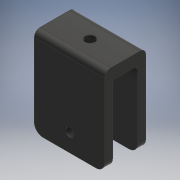
# Autodesk Inventor part: Y_Idler
Saved by Autodesk Inventor 2017.3 (Build 213256000, 256)
## iProperties
Created: 2018-09-09
Part Number: Y_Idler
Material: ABS Plastic
Document SubType Name: Modeling
Designer: Ax
Density: 1.06 g/cm^3
Appearance: Smooth - Black
Author: Ax
## iProperties of the stored document Y_Idler_3DPrint.ipt
Created: 2018-09-09
Part Number: Y_Idler_3DPrint
Material: Generic
Document SubType Name: Modeling
Designer: Ax
Density: 1 g/cm^3
Appearance: Default
Author: Ax
Autodesk Inventor part; units mm, degrees
ref_plane "YZ Plane" through (0, 0, 0) normal (1, 0, 0) x (0, 1, 0)
ref_plane "XZ Plane" through (0, 0, 0) normal (0, 1, 0) x (-1, 0, 0)
ref_plane "XY Plane" through (0, 0, 0) normal (0, 0, 1) x (1, 0, 0)
sketch "Sketch1" plane through (0, 0, 0) normal (1, 0, 0) x (0, 1, 0)
  line L0 (7, -26) -> (7, 4)
  line L1 (7, 4) -> (-7, 4)
  line L2 (-7, 4) -> (-7, -26)
  line L3 (-7, -26) -> (-4.25, -26)
  line L4 (-4.25, -26) -> (-4.25, 0)
  line L5 (-4.25, 0) -> (4.25, 0)
  line L6 (4.25, 0) -> (4.25, -26)
  line L7 (4.25, -26) -> (7, -26)
  line L8 (0, 0) -> (0, 4) construction
  dimension "d0" = 8.5
  dimension "d1" = 30
  dimension "d2" = 4
  dimension "d4" = 14
  constraints: 18 end point, 6 perpendicular, 2 equal length, 2 midpoint, 2 vertical, 1 coincident, 1 symmetric about line
  measures "d0" distance of L4.end L5.end
  measures "d1" distance of L0.start L0.end
  measures "d2" vertical distance of L0.end L5.end
  measures "d4" distance of L2.end L0.start
extrude "Extrusion1" add sketch "Sketch1" along normal mid plane 24
sketch "Sketch2" plane through (-12, 7, 4) normal (0, 1, 0) x (1, 0, 0)
  line L0 (12, 30) -> (12, 0) construction
  line L1 (24, 30) -> (0, 30) construction
  line L2 (0, 0) -> (24, 0) construction
  circle A0 centre (12, 24) radius 1.5
  point P0 (12, 4)
  dimension "d7" = 3
  dimension "d8" = 6
  constraints: 2 end point, 2 midpoint, 1 centre point, 1 point on line, 1 vertical
  measures "d7" diameter of A0
  measures "d8" distance of L0.start A0.centre
extrude "Extrusion2" cut sketch "Sketch2" against normal through all
sketch "Sketch3" plane through (-12, -7, 4) normal (0, 0, 1) x (1, 0, 0)
  circle A0 centre (12, 7) radius 1.7
  dimension "d11" = 3.4
  constraints: 1 centre point, 1 coincident
  measures "d11" diameter of A0
extrude "Extrusion3" cut sketch "Sketch3" against normal up to surface (4 mm away)
sketch "Sketch4" plane through (12, 4.25, 0) normal (0, 0, -1) x (-1, 0, 0)
  line L0 (15.2909, -4.25) -> (13.6454, -7.1)
  line L1 (13.6454, -7.1) -> (10.3546, -7.1)
  line L2 (10.3546, -7.1) -> (8.7091, -4.25)
  line L3 (8.7091, -4.25) -> (10.3546, -1.4)
  line L4 (10.3546, -1.4) -> (13.6454, -1.4)
  line L5 (13.6454, -1.4) -> (15.2909, -4.25)
  point P0 (12, -4.25)
  point P1 (12, -4.25)
  dimension "d14" = 5.7
  constraints: 12 end point, 1 coincident, 1 horizontal, 13 other
  measures "d14" distance of L4.end L0.end
extrude "Extrusion4" cut sketch "Sketch4" against normal blind 3
fillet "Fillet1" radius 2 2 edges at (0, 7, 4) (0, -7, 4)
fillet "Fillet2" radius 3 4 edges at (12, -5.625, -26) (12, 5.625, -26) (-12, 5.625, -26) (-12, -5.625, -26)
fillet "Fillet3" radius 1 2 edges at (0, 4.25, 0) (0, -4.25, 0)
body "Solid1"
